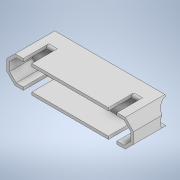
# Autodesk Inventor part: Magazin_Stössel
Saved by Autodesk Inventor 2021 (Build 250183000, 183)
## iProperties
Created: 2024-05-14
Part Number: Magazin_Stössel
Material: Generic
Document SubType Name: Modeling
Designer: Lukas
Density: 1 g/cm^3
Appearance: Default
Author: Lukas
Autodesk Inventor part; units mm, degrees
ref_plane "YZ Plane" through (0, 0, 0) normal (1, 0, 0) x (0, 1, 0)
ref_plane "XZ Plane" through (0, 0, 0) normal (0, 1, 0) x (-1, 0, 0)
ref_plane "XY Plane" through (0, 0, 0) normal (0, 0, 1) x (1, 0, 0)
sketch "Sketch1" plane through (0, 0, 0) normal (0, 0, 1) x (1, 0, 0)
  line L0 (-22.5, 2) -> (-19.5, 5)
  line L1 (-19.5, 5) -> (19.5, 5)
  line L2 (19.5, 5) -> (22.5, 2)
  line L3 (22.5, 2) -> (22.5, -2)
  line L4 (22.5, -2) -> (19.5, -5)
  line L5 (19.5, -5) -> (-19.5, -5)
  line L6 (-19.5, -5) -> (-22.5, -2)
  line L7 (-22.5, -2) -> (-22.5, 2)
  line L8 (19.4379, 4.85) -> (-19.4379, 4.85)
  line L9 (-19.4379, 4.85) -> (-22.35, 1.9379)
  line L10 (-22.35, 1.9379) -> (-22.35, -1.9379)
  line L11 (-22.35, -1.9379) -> (-19.4379, -4.85)
  line L12 (-19.4379, -4.85) -> (19.4379, -4.85)
  line L13 (19.4379, -4.85) -> (22.35, -1.9379)
  line L14 (22.35, -1.9379) -> (22.35, 1.9379)
  line L15 (22.35, 1.9379) -> (19.4379, 4.85)
  point P0 (0, 0)
  point P1 (0, 5)
  point P2 (-22.5, 0)
  dimension "d0" = 3
  dimension "d1" = 3
  dimension "d2" = 10
  dimension "d3" = 39
  dimension "d4" = 0.15
  constraints: 32 end point, 9 perpendicular, 4 parallel, 2 midpoint, 2 vertical alignment, 1 horizontal, 1 horizontal alignment, 7 other
  measures "d0" horizontal distance of L0.start L0.end
  measures "d1" horizontal distance of L0.start L0.end
  measures "d2" distance between parallel lines of L5 L1
  measures "d3" distance of L0.end L1.end
  measures "d4" distance between parallel lines of L1 L8
extrude "Extrusion1" add sketch "Sketch1" along normal blind 14 contours L15 L14 L13 L12 L11 L10 L9 L8
sketch "Sketch2" plane through (-22.35, -1.9379, 0) normal (-1, 0, 0) x (0, 0, 1)
  circle A0 centre (0, 1.9379) radius 4.5
  dimension "d7" = 9
  constraints: 1 centre point, 1 coincident
  measures "d7" diameter of A0
extrude "Extrusion2" cut sketch "Sketch2" against normal through all
sketch "Sketch3" plane through (0, 0, 14) normal (0, 0, 1) x (1, 0, 0)
  line L0 (-19.4379, 4.85) -> (-22.35, 1.9379) projected
  line L1 (-22.35, 1.9379) -> (-22.35, -1.9379) projected
  line L2 (-22.35, -1.9379) -> (-19.4379, -4.85) projected
  line L3 (-19.4379, -4.85) -> (19.4379, -4.85) projected
  line L4 (19.4379, -4.85) -> (22.35, -1.9379) projected
  line L5 (22.35, -1.9379) -> (22.35, 1.9379) projected
  line L6 (22.35, 1.9379) -> (19.4379, 4.85) projected
  line L7 (19.4379, 4.85) -> (-19.4379, 4.85) projected
  line L8 (-19.0237, 3.85) -> (-21.35, 1.5237)
  line L9 (-21.35, 1.5237) -> (-21.35, -1.5237)
  line L10 (-21.35, -1.5237) -> (-19.0237, -3.85)
  line L11 (-19.0237, -3.85) -> (19.0237, -3.85)
  line L12 (19.0237, -3.85) -> (21.35, -1.5237)
  line L13 (21.35, -1.5237) -> (21.35, 1.5237)
  line L14 (21.35, 1.5237) -> (19.0237, 3.85)
  line L15 (19.0237, 3.85) -> (-19.0237, 3.85)
  line L16 (19.4379, 4.85) -> (-19.4379, 4.85) projected
  line L17 (-16.5, 3.85) -> (-13.5, 3.85)
  line L18 (-13.5, 3.85) -> (-13.5, 4.85)
  line L19 (-13.5, 4.85) -> (-16.5, 4.85)
  line L20 (-16.5, 4.85) -> (-16.5, 3.85)
  line L21 (-19.4379, -4.85) -> (19.4379, -4.85) projected
  line L22 (-16.5, -4.85) -> (-13.5, -4.85)
  line L23 (-13.5, -4.85) -> (-13.5, -3.85)
  line L24 (-13.5, -3.85) -> (-16.5, -3.85)
  line L25 (-16.5, -3.85) -> (-16.5, -4.85)
  line L26 (13.5, -3.85) -> (16.5, -3.85)
  line L27 (16.5, -3.85) -> (16.5, -4.85)
  line L28 (16.5, -4.85) -> (13.5, -4.85)
  line L29 (13.5, -4.85) -> (13.5, -3.85)
  line L30 (13.5, 3.85) -> (16.5, 3.85)
  line L31 (16.5, 3.85) -> (16.5, 4.85)
  line L32 (16.5, 4.85) -> (13.5, 4.85)
  line L33 (13.5, 4.85) -> (13.5, 3.85)
  point P0 (0, 0)
  point P1 (13.5, 4.85)
  point P2 (16.5, 3.85)
  point P3 (16.5, -3.85)
  point P4 (-16.5, -3.85)
  point P5 (-13.5, 3.85)
  dimension "d10" = 1
  dimension "d15" = 3
  dimension "d16" = 3
  dimension "d18" = 5.85
  dimension "d19" = 5.85
  constraints: 48 end point, 12 point on line, 8 parallel, 4 horizontal, 4 perpendicular, 7 other
  measures "d10" distance between parallel lines of L7 L15
  measures "d15" distance between parallel lines of L18 L20
  measures "d16" distance from line of L30.start L31
  measures "d18" distance between parallel lines of L20 L1
  measures "d19" distance between parallel lines of L5 L31
extrude "Extrusion3" cut sketch "Sketch3" against normal blind 8 contours L7 L18 L15 L20 | L15 L14 L13 L12 L11 L10 L9 L8 | L7 L31 L15 L33 | L25 L11 L23 L3 | L29 L11 L27 L3
fillet "Fillet1" radius 1 4 edges at (-15, 4.85, 6) (15, 4.85, 6) (15, -4.85, 6) (-15, -4.85, 6)
equation "\"d16\" = d15"
equation "\"d19\" = d18"
body "Solid1"
